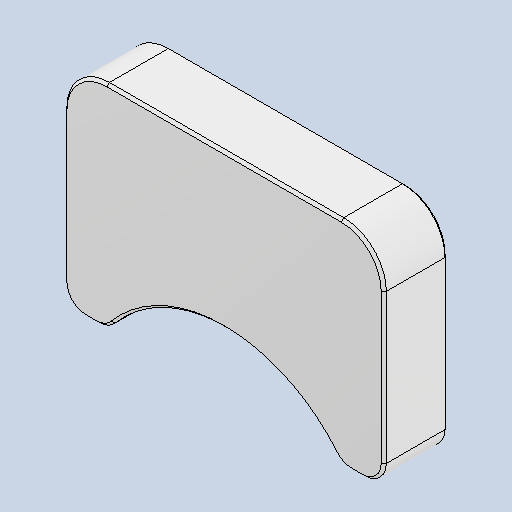
# Autodesk Inventor part: pld-pip-support
Saved by Autodesk Inventor 2026 (Build 300175050, 175E)
## iProperties
Created: 2025-11-14
Part Number: pld-pip-support
Material: ABS Plastic
Document SubType Name: Modeling
Designer: kuzmin
Density: 1.06 g/cm^3
Appearance: Smooth - White
Author: kuzmin
Autodesk Inventor part; units mm, degrees
ref_plane "YZ Plane" through (0, 0, 0) normal (1, 0, 0) x (0, 1, 0)
ref_plane "XZ Plane" through (0, 0, 0) normal (0, 1, 0) x (-1, 0, 0)
ref_plane "XY Plane" through (0, 0, 0) normal (0, 0, 1) x (1, 0, 0)
sketch "Sketch1" plane through (0, 0, 0) normal (0, 0, 1) x (-1, 0, 0)
  line L0 (-37.5, 50) -> (37.5, 50)
  line L1 (37.5, 50) -> (37.5, 0)
  line L2 (37.5, 0) -> (-37.5, 0)
  line L3 (-37.5, 0) -> (-37.5, 50)
  arc A0 (-27.5, 50) -> (27.5, 50) centre (0, 69.9937) ccw
  point P0 (0, 0)
  point P1 (0, 0)
  dimension "d1" = 68
  dimension "d2" = 50
  dimension "d4" = 75
  dimension "d5" = 10
  constraints: 8 end point, 2 parallel, 2 point on circle, 2 point on line, 1 centre point, 1 coincident, 1 horizontal, 1 midpoint, 1 perpendicular, 1 vertical alignment
  measures "d1" diameter of A0
  measures "d2" distance of L0.end L1.end
  measures "d4" distance of L1.end L2.end
  measures "d5" distance of L0.end A0.end
extrude "Extrusion1" add sketch "Sketch1" along normal blind 15 contours L0 A0 L1 L2 L3
fillet "Fillet1" radius 10 2 edges at (37.5, 0, 7.5) (-37.5, 0, 7.5)
fillet "Fillet2" radius 5 4 edges at (-27.5, -50, 7.5) (-37.5, -50, 7.5) (27.5, -50, 7.5) (37.5, -50, 7.5)
chamfer "Chamfer1" distance 0.6 angle 45 24 edges at (0, -35.9937, 15) (27.8197, -49.5289, 15) (31.2192, -50, 15) (36.0355, -48.5355, 15) (37.5, -27.5, 15) (34.5711, -2.9289, 15) (0, 0, 15) (-34.5711, -2.9289, 15) (-37.5, -27.5, 15) (-36.0355, -48.5355, 15) (-31.2192, -50, 15) (-27.8197, -49.5289, 15) (0, -35.9937, 0) (27.8197, -49.5289, 0) (31.2192, -50, 0) (36.0355, -48.5355, 0) (37.5, -27.5, 0) (34.5711, -2.9289, 0) (0, 0, 0) (-34.5711, -2.9289, 0) (-37.5, -27.5, 0) (-36.0355, -48.5355, 0) (-31.2192, -50, 0) (-27.8197, -49.5289, 0)
body "Solid1"
